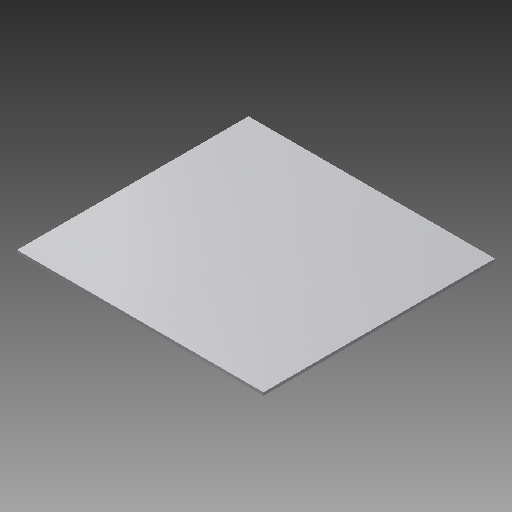
# Autodesk Inventor part: PVC_Bodenplatte_schwarz
Saved by Autodesk Inventor 2018 (Build 220112000, 112)
## iProperties
Created: 2012-11-14
Part Number: PVC_Bodenplatte_schwarz
Material: PVC-U
Document SubType Name: Modeling
Designer: Neef
Mass: 4222.94 g
Surface Area: 8388.8 cm^2
Volume: 3273.6 cm^3
Density: 1.29 g/cm^3
Appearance: Smooth - White
Author: Neef
Autodesk Inventor part; units mm, degrees
ref_plane "YZ Plane" through (0, 0, 0) normal (1, 0, 0) x (0, 1, 0)
ref_plane "XZ Plane" through (0, 0, 0) normal (0, 1, 0) x (-1, 0, 0)
ref_plane "XY Plane" through (0, 0, 0) normal (0, 0, 1) x (1, 0, 0)
sketch "Skizze1" plane through (0, 0, 0) normal (0, 0, 1) x (1, 0, 0)
  line L0 (0, 434) -> (0, -434) projected
  line L1 (-462, 0) -> (462, 0) projected
  line L2 (330, -310) -> (-330, -310)
  line L3 (-330, -310) -> (-330, 310)
  line L4 (-330, 310) -> (330, 310)
  line L5 (330, 310) -> (330, -310)
  point P0 (0, 0)
  point P1 (0, -310)
  point P2 (-330, 0)
  dimension "d0" = 660
  dimension "d1" = 620
  constraints: 8 end point, 2 midpoint, 2 parallel, 2 point on line, 1 horizontal, 1 perpendicular
  measures "d0" distance of L2.start L2.end
  measures "d1" distance of L2.end L3.end
extrude "Extrusion1" add sketch "Skizze1" along normal blind 8
